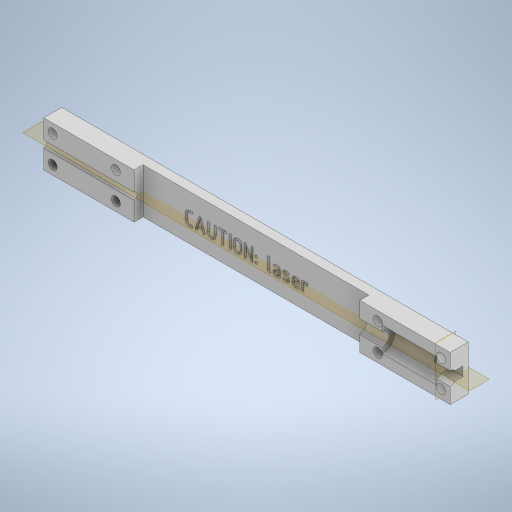
# Autodesk Inventor part: common_bottom
Saved by Autodesk Inventor 2024 (Build 280153000, 153)
## iProperties
Created: 2023-10-30
Part Number: common_bottom
Material: Generic
Document SubType Name: Modeling
Designer: toybox
Density: 1 g/cm^3
Appearance: Default
Author: toybox
Autodesk Inventor part; units mm, degrees
ref_plane "YZ Plane" through (0, 0, 0) normal (1, 0, 0) x (0, 1, 0)
ref_plane "XZ Plane" through (0, 0, 0) normal (0, 1, 0) x (-1, 0, 0)
ref_plane "XY Plane" through (0, 0, 0) normal (0, 0, 1) x (1, 0, 0)
sketch "Sketch1" plane through (0, 0, 0) normal (0, 0, 1) x (1, 0, 0)
  line L0 (-45, 5) -> (45, 5)
  line L1 (45, 5) -> (45, -5)
  line L2 (45, -5) -> (-45, -5)
  line L3 (-45, -5) -> (-45, 5)
  line L4 (-45, 5) -> (45, -5) construction
  line L5 (45, 5) -> (-45, -5) construction
  point P0 (0, 0)
  dimension "d0" = 90
  dimension "d1" = 10
  constraints: 12 end point, 2 midpoint, 2 parallel, 1 horizontal, 1 perpendicular
  measures "d0" distance of L1.end L2.end
  measures "d1" distance of L0.end L1.end
extrude "Extrusion1" add sketch "Sketch1" along normal blind 2
sketch "Sketch4" plane through (0, 0, 2) normal (0, 0, 1) x (1, 0, 0)
  line L0 (45, -5) -> (45, 5) projected
  line L1 (-45, -5) -> (45, -5) projected
  line L2 (45, 5) -> (25, 5)
  line L3 (25, 5) -> (25, -5)
  line L4 (25, -5) -> (45, -5)
  line L5 (45, -5) -> (45, 5)
  line L6 (45, 5) -> (-45, 5) projected
  line L7 (-45, 5) -> (-25, 5)
  line L8 (-25, 5) -> (-25, -5)
  line L9 (-25, -5) -> (-45, -5)
  line L10 (-45, -5) -> (-45, 5)
  point P0 (0, 0)
  dimension "d13" = 20
  dimension "d14" = 20
  constraints: 16 end point, 4 parallel, 2 horizontal, 2 perpendicular, 2 point on line
  measures "d13" distance of L4.end L3.end
  measures "d14" distance of L8.end L9.end
extrude "Extrusion4" add sketch "Sketch4" along normal blind 2 contours L1 L3 L2 L0 | L1 L10 L6 L8
sketch "Sketch5" plane through (0, 0, 4) normal (0, 0, 1) x (1, 0, 0)
  circle A0 centre (43, 3) radius 1
  circle A1 centre (43, -3) radius 1
  circle A2 centre (-43.0005, -3) radius 1
  circle A3 centre (-43.0005, 3) radius 1
  circle A4 centre (-28.9998, -3) radius 1
  circle A5 centre (-28.9998, 3) radius 1
  circle A6 centre (28.9998, -3) radius 1
  circle A7 centre (28.9998, 3) radius 1
  point P0 (0, 0)
  dimension "d17" = 2
  dimension "d18" = 2
  dimension "d19" = 2
  dimension "d20" = 2
  dimension "d22" = 2
  dimension "d23" = 2
  dimension "d24" = 2
  dimension "d25" = 2
  constraints: 8 centre point
  measures "d17" diameter of A0
  measures "d18" diameter of A1
  measures "d19" diameter of A2
  measures "d20" diameter of A3
  measures "d22" diameter of A4
  measures "d23" diameter of A5
  measures "d24" diameter of A6
  measures "d25" diameter of A7
extrude "Extrusion5" cut sketch "Sketch5" against normal through all
sketch "Sketch6" plane through (45, -5, 0) normal (1, 0, 0) x (0, 0, -1)
  line L0 (-4, 0) -> (-4, 10) projected
  circle A0 centre (-4, 5) radius 1.5
  point P0 (0, 5)
  point P1 (-4, 6.5)
  point P2 (-4, 3.5)
  dimension "d28" = 3
  constraints: 1 centre point, 1 midpoint
  measures "d28" diameter of A0
extrude "Extrusion6" cut sketch "Sketch6" against normal blind 20 contours L0 A0 picked at (-3.6883, 5.3909)
sketch "Sketch7" plane through (-45, -5, 0) normal (-1, 0, 0) x (0, 0, 1)
  line L0 (4, 0) -> (4, 10) projected
  circle A0 centre (4, 5) radius 0.75
  point P0 (0, 5)
  dimension "d31" = 1.5
  constraints: 1 centre point, 1 midpoint
  measures "d31" diameter of A0
extrude "Extrusion7" cut sketch "Sketch7" against normal blind 20
ref_plane "Work Plane1" through (42, -5, 0) normal (1, 0, 0) x (0, 0, -1)
sketch "Sketch8" plane through (42, -5, 0) normal (1, 0, 0) x (0, 0, -1)
  arc A0 (-4, 3.5) -> (-4, 6.5) centre (-4, 5) ccw projected
  circle A1 centre (-4, 5) radius 2.7
  point P0 (0, 5)
  dimension "d35" = 5.4
  constraints: 1 centre point, 1 coincident
  measures "d35" diameter of A1
extrude "Extrusion8" cut sketch "Sketch8" against normal blind 12
ref_plane "Work Plane3" through (-45, 0, 0) normal (0, 1, 0) x (1, 0, 0)
sketch "Sketch10" plane through (-45, 0, 0) normal (0, 1, 0) x (1, 0, 0)
  line L0 (90, -2.5) -> (90, -4) projected
  line L1 (90, -4) -> (84, -4)
  line L2 (84, -4) -> (84, -1.2)
  line L3 (84, -1.2) -> (90, -1.2)
  line L4 (90, -1.2) -> (90, -4)
  point P0 (45, 0)
  dimension "d42" = 6
  dimension "d43" = 2.8
  constraints: 8 end point, 2 parallel, 1 horizontal, 1 perpendicular
  measures "d42" distance of L2.end L3.end
  measures "d43" distance of L1.end L2.end
extrude "Extrusion10" cut sketch "Sketch10" along normal mid plane 2
sketch "Sketch11" plane through (0, 0, 2) normal (0, 0, 1) x (1, 0, 0)
  line L0 (-15.8496, 1.3732) -> (11.6508, 1.3732) construction
  line L1 (11.6508, 1.3732) -> (11.6508, -1.6796) construction
  line L2 (11.6508, -1.6796) -> (-15.8496, -1.6796) construction
  line L3 (-15.8496, -1.6796) -> (-15.8496, 1.3732) construction
  spline S0 degree 2 poles (-14.1747, 1.3732) (-13.9787, 1.3732) (-13.9787, 1.18) knots 0 0 0 1 1 1
  spline S1 degree 2 poles (-13.9787, 1.18) (-13.9787, 0.9839) (-14.1747, 0.9839) knots 0 0 0 1 1 1
  line L4 (-14.1747, 0.9839) -> (-14.7685, 0.9839)
  spline S2 degree 2 poles (-14.7685, 0.9839) (-14.9337, 0.9839) (-15.1634, 0.7515) (-15.1634, 0.589) knots 0 0 0 1 2 2 2
  line L5 (-15.1634, 0.589) -> (-15.1634, -0.8925)
  spline S3 degree 2 poles (-15.1634, -0.8925) (-15.1634, -1.0578) (-14.9309, -1.2903) (-14.7685, -1.2903) knots 0 0 0 1 2 2 2
  line L6 (-14.7685, -1.2903) -> (-14.1747, -1.2903)
  spline S4 degree 2 poles (-14.1747, -1.2903) (-13.9787, -1.2903) (-13.9787, -1.4835) knots 0 0 0 1 1 1
  spline S5 degree 2 poles (-13.9787, -1.4835) (-13.9787, -1.6796) (-14.1747, -1.6796) knots 0 0 0 1 1 1
  line L7 (-14.1747, -1.6796) -> (-14.7685, -1.6796)
  spline S6 degree 2 poles (-14.7685, -1.6796) (-15.0962, -1.6796) (-15.5555, -1.2202) (-15.5555, -0.8925) knots 0 0 0 1 2 2 2
  line L8 (-15.5555, -0.8925) -> (-15.5555, 0.589)
  spline S7 degree 2 poles (-15.5555, 0.589) (-15.5555, 0.9139) (-15.0962, 1.3732) (-14.7685, 1.3732) knots 0 0 0 1 2 2 2
  line L9 (-14.7685, 1.3732) -> (-14.1747, 1.3732)
  spline S8 degree 2 poles (-11.2732, -1.4835) (-11.2732, -1.6796) (-11.4692, -1.6796) knots 0 0 0 1 1 1
  spline S9 degree 2 poles (-11.4692, -1.6796) (-11.6121, -1.6796) (-11.6541, -1.5479) knots 0 0 0 1 1 1
  line L10 (-11.6541, -1.5479) -> (-11.8585, -0.9402)
  line L11 (-11.8585, -0.9402) -> (-12.8556, -0.9402)
  line L12 (-12.8556, -0.9402) -> (-13.0572, -1.5479)
  spline S10 degree 2 poles (-13.0572, -1.5479) (-13.102, -1.6796) (-13.2449, -1.6796) knots 0 0 0 1 1 1
  spline S11 degree 2 poles (-13.2449, -1.6796) (-13.4381, -1.6796) (-13.4381, -1.4835) knots 0 0 0 1 1 1
  spline S12 degree 2 poles (-13.4381, -1.4835) (-13.4381, -1.4499) (-13.4297, -1.4219) knots 0 0 0 1 1 1
  line L13 (-13.4297, -1.4219) -> (-12.5503, 1.222)
  spline S13 degree 2 poles (-12.5503, 1.222) (-12.4999, 1.3704) (-12.357, 1.3704) knots 0 0 0 1 1 1
  spline S14 degree 2 poles (-12.357, 1.3704) (-12.2142, 1.3704) (-12.1666, 1.2248) knots 0 0 0 1 1 1
  line L14 (-12.1666, 1.2248) -> (-11.2816, -1.4219)
  spline S15 degree 2 poles (-11.2816, -1.4219) (-11.2732, -1.4527) (-11.2732, -1.4835) knots 0 0 0 1 1 1
  line L15 (-12.357, 0.6619) -> (-12.7436, -0.5509)
  line L16 (-12.7436, -0.5509) -> (-11.9677, -0.5509)
  line L17 (-11.9677, -0.5509) -> (-12.357, 0.6619)
  line L18 (-8.8505, 1.1772) -> (-8.8505, -0.7441)
  spline S16 degree 2 poles (-8.8505, -0.7441) (-8.8505, -1.1334) (-9.3967, -1.6796) (-9.7832, -1.6796) knots 0 0 0 1 2 2 2
  spline S17 degree 2 poles (-9.7832, -1.6796) (-10.1725, -1.6796) (-10.7186, -1.1334) (-10.7186, -0.7441) knots 0 0 0 1 2 2 2
  line L19 (-10.7186, -0.7441) -> (-10.7186, 1.1772)
  spline S18 degree 2 poles (-10.7186, 1.1772) (-10.7186, 1.3704) (-10.5226, 1.3704) knots 0 0 0 1 1 1
  spline S19 degree 2 poles (-10.5226, 1.3704) (-10.3265, 1.3704) (-10.3265, 1.1772) knots 0 0 0 1 1 1
  line L20 (-10.3265, 1.1772) -> (-10.3265, -0.7441)
  spline S20 degree 2 poles (-10.3265, -0.7441) (-10.3265, -0.9738) (-10.0128, -1.2903) (-9.7832, -1.2903) knots 0 0 0 1 2 2 2
  spline S21 degree 2 poles (-9.7832, -1.2903) (-9.5563, -1.2903) (-9.2426, -0.9738) (-9.2426, -0.7441) knots 0 0 0 1 2 2 2
  line L21 (-9.2426, -0.7441) -> (-9.2426, 1.1772)
  spline S22 degree 2 poles (-9.2426, 1.1772) (-9.2426, 1.3704) (-9.0466, 1.3704) knots 0 0 0 1 1 1
  spline S23 degree 2 poles (-9.0466, 1.3704) (-8.8505, 1.3704) (-8.8505, 1.1772) knots 0 0 0 1 1 1
  spline S24 degree 2 poles (-8.3016, 1.18) (-8.3016, 1.3732) (-8.1055, 1.3732) knots 0 0 0 1 1 1
  line L22 (-8.1055, 1.3732) -> (-6.6267, 1.3732)
  spline S25 degree 2 poles (-6.6267, 1.3732) (-6.4307, 1.3732) (-6.4307, 1.18) knots 0 0 0 1 1 1
  spline S26 degree 2 poles (-6.4307, 1.18) (-6.4307, 0.9839) (-6.6267, 0.9839) knots 0 0 0 1 1 1
  line L23 (-6.6267, 0.9839) -> (-7.1701, 0.9839)
  line L24 (-7.1701, 0.9839) -> (-7.1701, -1.4835)
  spline S27 degree 2 poles (-7.1701, -1.4835) (-7.1701, -1.6796) (-7.3661, -1.6796) knots 0 0 0 1 1 1
  spline S28 degree 2 poles (-7.3661, -1.6796) (-7.5622, -1.6796) (-7.5622, -1.4835) knots 0 0 0 1 1 1
  line L25 (-7.5622, -1.4835) -> (-7.5622, 0.9839)
  line L26 (-7.5622, 0.9839) -> (-8.1055, 0.9839)
  spline S29 degree 2 poles (-8.1055, 0.9839) (-8.3016, 0.9839) (-8.3016, 1.18) knots 0 0 0 1 1 1
  spline S30 degree 2 poles (-5.6913, -1.6796) (-5.8874, -1.6796) (-5.8874, -1.4835) knots 0 0 0 1 1 1
  line L27 (-5.8874, -1.4835) -> (-5.8874, 1.1772)
  spline S31 degree 2 poles (-5.8874, 1.1772) (-5.8874, 1.3704) (-5.6913, 1.3704) knots 0 0 0 1 1 1
  spline S32 degree 2 poles (-5.6913, 1.3704) (-5.4952, 1.3704) (-5.4952, 1.1772) knots 0 0 0 1 1 1
  line L28 (-5.4952, 1.1772) -> (-5.4952, -1.4835)
  spline S33 degree 2 poles (-5.4952, -1.4835) (-5.4952, -1.6796) (-5.6913, -1.6796) knots 0 0 0 1 1 1
  spline S34 degree 2 poles (-3.109, -0.7441) (-3.109, -1.1306) (-3.6552, -1.6796) (-4.0417, -1.6796) knots 0 0 0 1 2 2 2
  spline S35 degree 2 poles (-4.0417, -1.6796) (-4.431, -1.6796) (-4.9771, -1.1334) (-4.9771, -0.7441) knots 0 0 0 1 2 2 2
  line L29 (-4.9771, -0.7441) -> (-4.9771, 0.4406)
  spline S36 degree 2 poles (-4.9771, 0.4406) (-4.9771, 0.8271) (-4.431, 1.3732) (-4.0417, 1.3732) knots 0 0 0 1 2 2 2
  spline S37 degree 2 poles (-4.0417, 1.3732) (-3.6524, 1.3732) (-3.109, 0.8271) (-3.109, 0.4406) knots 0 0 0 1 2 2 2
  line L30 (-3.109, 0.4406) -> (-3.109, -0.7441)
  line L31 (-3.5011, -0.7441) -> (-3.5011, 0.4406)
  spline S38 degree 2 poles (-3.5011, 0.4406) (-3.5011, 0.6675) (-3.8148, 0.9839) (-4.0417, 0.9839) knots 0 0 0 1 2 2 2
  spline S39 degree 2 poles (-4.0417, 0.9839) (-4.2713, 0.9839) (-4.585, 0.6675) (-4.585, 0.4406) knots 0 0 0 1 2 2 2
  line L32 (-4.585, 0.4406) -> (-4.585, -0.7441)
  spline S40 degree 2 poles (-4.585, -0.7441) (-4.585, -0.9738) (-4.2713, -1.2903) (-4.0417, -1.2903) knots 0 0 0 1 2 2 2
  spline S41 degree 2 poles (-4.0417, -1.2903) (-3.8148, -1.2903) (-3.5011, -0.9738) (-3.5011, -0.7441) knots 0 0 0 1 2 2 2
  line L33 (-1.0841, -0.8645) -> (-1.0841, 1.1772)
  spline S42 degree 2 poles (-1.0841, 1.1772) (-1.0841, 1.3704) (-0.888, 1.3704) knots 0 0 0 1 1 1
  spline S43 degree 2 poles (-0.888, 1.3704) (-0.692, 1.3704) (-0.692, 1.1772) knots 0 0 0 1 1 1
  line L34 (-0.692, 1.1772) -> (-0.692, -1.4835)
  spline S44 degree 2 poles (-0.692, -1.4835) (-0.692, -1.6796) (-0.888, -1.6796) knots 0 0 0 1 1 1
  spline S45 degree 2 poles (-0.888, -1.6796) (-1.0085, -1.6796) (-1.0617, -1.5815) knots 0 0 0 1 1 1
  line L35 (-1.0617, -1.5815) -> (-2.168, 0.561)
  line L36 (-2.168, 0.561) -> (-2.168, -1.4835)
  spline S46 degree 2 poles (-2.168, -1.4835) (-2.168, -1.6796) (-2.364, -1.6796) knots 0 0 0 1 1 1
  spline S47 degree 2 poles (-2.364, -1.6796) (-2.5601, -1.6796) (-2.5601, -1.4835) knots 0 0 0 1 1 1
  line L37 (-2.5601, -1.4835) -> (-2.5601, 1.1772)
  spline S48 degree 2 poles (-2.5601, 1.1772) (-2.5601, 1.3704) (-2.364, 1.3704) knots 0 0 0 1 1 1
  spline S49 degree 2 poles (-2.364, 1.3704) (-2.2492, 1.3704) (-2.2016, 1.2864) knots 0 0 0 1 1 1
  line L38 (-2.2016, 1.2864) -> (-1.0841, -0.8645)
  spline S50 degree 2 poles (-0.1458, -1.1866) (-0.1458, -0.9962) (0.0502, -0.9962) knots 0 0 0 1 1 1
  spline S51 degree 2 poles (0.0502, -0.9962) (0.2463, -0.9962) (0.2463, -1.1866) knots 0 0 0 1 1 1
  line L39 (0.2463, -1.1866) -> (0.2463, -1.3351)
  spline S52 degree 2 poles (0.2463, -1.3351) (0.2463, -1.5311) (0.0502, -1.5311) knots 0 0 0 1 1 1
  spline S53 degree 2 poles (0.0502, -1.5311) (-0.1458, -1.5311) (-0.1458, -1.3351) knots 0 0 0 1 1 1
  line L40 (-0.1458, -1.3351) -> (-0.1458, -1.1866)
  spline S54 degree 2 poles (-0.1458, -0.0047) (-0.1458, 0.1885) (0.0502, 0.1885) knots 0 0 0 1 1 1
  spline S55 degree 2 poles (0.0502, 0.1885) (0.2463, 0.1885) (0.2463, -0.0047) knots 0 0 0 1 1 1
  line L41 (0.2463, -0.0047) -> (0.2463, -0.1532)
  spline S56 degree 2 poles (0.2463, -0.1532) (0.2463, -0.3464) (0.0502, -0.3464) knots 0 0 0 1 1 1
  spline S57 degree 2 poles (0.0502, -0.3464) (-0.1458, -0.3464) (-0.1458, -0.1532) knots 0 0 0 1 1 1
  line L42 (-0.1458, -0.1532) -> (-0.1458, -0.0047)
  spline S58 degree 2 poles (2.5765, 1.1772) (2.5765, 1.3704) (2.7725, 1.3704) knots 0 0 0 1 1 1
  spline S59 degree 2 poles (2.7725, 1.3704) (2.9686, 1.3704) (2.9686, 1.1772) knots 0 0 0 1 1 1
  line L43 (2.9686, 1.1772) -> (2.9686, -1.1894)
  spline S60 degree 2 poles (2.9686, -1.1894) (2.9686, -1.2678) (3.2654, -1.3351) (3.2654, -1.4835) knots 0 0 0 1 2 2 2
  spline S61 degree 2 poles (3.2654, -1.4835) (3.2654, -1.6796) (3.0694, -1.6796) knots 0 0 0 1 1 1
  spline S62 degree 2 poles (3.0694, -1.6796) (2.8481, -1.6796) (2.5765, -1.4191) (2.5765, -1.1894) knots 0 0 0 1 2 2 2
  line L44 (2.5765, -1.1894) -> (2.5765, 1.1772)
  spline S63 degree 2 poles (4.4278, -1.6796) (4.1561, -1.6796) (3.7864, -1.3099) (3.7864, -1.0382) knots 0 0 0 1 2 2 2
  spline S64 degree 2 poles (3.7864, -1.0382) (3.7864, -0.8673) (3.8732, -0.7189) knots 0 0 0 1 1 1
  spline S65 degree 2 poles (3.8732, -0.7189) (4.0525, -0.4024) (4.4278, -0.4024) knots 0 0 0 1 1 1
  line L45 (4.4278, -0.4024) -> (4.9711, -0.4024)
  line L46 (4.9711, -0.4024) -> (4.9711, -0.1504)
  spline S66 degree 2 poles (4.9711, -0.1504) (4.9711, -0.0467) (4.8283, 0.0961) (4.7218, 0.0961) knots 0 0 0 1 2 2 2
  line L47 (4.7218, 0.0961) -> (4.1309, 0.0961)
  spline S67 degree 2 poles (4.1309, 0.0961) (3.9348, 0.0961) (3.9348, 0.2922) knots 0 0 0 1 1 1
  spline S68 degree 2 poles (3.9348, 0.2922) (3.9348, 0.4854) (4.1309, 0.4854) knots 0 0 0 1 1 1
  line L48 (4.1309, 0.4854) -> (4.7218, 0.4854)
  spline S69 degree 2 poles (4.7218, 0.4854) (4.9907, 0.4854) (5.3632, 0.1157) (5.3632, -0.1504) knots 0 0 0 1 2 2 2
  line L49 (5.3632, -0.1504) -> (5.3632, -1.4835)
  spline S70 degree 2 poles (5.3632, -1.4835) (5.3632, -1.6796) (5.1671, -1.6796) knots 0 0 0 1 1 1
  line L50 (5.1671, -1.6796) -> (4.4278, -1.6796)
  line L51 (4.9711, -0.7917) -> (4.4278, -0.7917)
  spline S71 degree 2 poles (4.4278, -0.7917) (4.3241, -0.7917) (4.1785, -0.9374) (4.1785, -1.0382) knots 0 0 0 1 2 2 2
  spline S72 degree 2 poles (4.1785, -1.0382) (4.1785, -1.1418) (4.3269, -1.2903) (4.4278, -1.2903) knots 0 0 0 1 2 2 2
  line L52 (4.4278, -1.2903) -> (4.9711, -1.2903)
  line L53 (4.9711, -1.2903) -> (4.9711, -0.7917)
  spline S73 degree 2 poles (7.0857, -1.1138) (7.0857, -1.0018) (6.9876, -0.9542) knots 0 0 0 1 1 1
  line L54 (6.9876, -0.9542) -> (6.2286, -0.5901)
  spline S74 degree 2 poles (6.2286, -0.5901) (5.9037, -0.4332) (5.9037, -0.0775) knots 0 0 0 1 1 1
  spline S75 degree 2 poles (5.9037, -0.0775) (5.9037, 0.2025) (6.1334, 0.3538) knots 0 0 0 1 1 1
  spline S76 degree 2 poles (6.1334, 0.3538) (6.3267, 0.4826) (6.6151, 0.4826) knots 0 0 0 1 1 1
  spline S77 degree 2 poles (6.6151, 0.4826) (6.9568, 0.4826) (7.2285, 0.3118) knots 0 0 0 1 1 1
  spline S78 degree 2 poles (7.2285, 0.3118) (7.3293, 0.2474) (7.3293, 0.1437) knots 0 0 0 1 1 1
  spline S79 degree 2 poles (7.3293, 0.1437) (7.3293, 0.0625) (7.2145, -0.0523) (7.1333, -0.0523) knots 0 0 0 1 2 2 2
  spline S80 degree 2 poles (7.1333, -0.0523) (7.08, -0.0523) (7.0156, -0.0131) knots 0 0 0 1 1 1
  spline S81 degree 2 poles (7.0156, -0.0131) (6.8392, 0.0933) (6.6151, 0.0933) knots 0 0 0 1 1 1
  spline S82 degree 2 poles (6.6151, 0.0933) (6.293, 0.0933) (6.293, -0.0775) knots 0 0 0 1 1 1
  spline S83 degree 2 poles (6.293, -0.0775) (6.293, -0.1924) (6.3883, -0.2372) knots 0 0 0 1 1 1
  line L55 (6.3883, -0.2372) -> (7.1529, -0.6069)
  spline S84 degree 2 poles (7.1529, -0.6069) (7.4778, -0.7637) (7.4778, -1.1138) knots 0 0 0 1 1 1
  spline S85 degree 2 poles (7.4778, -1.1138) (7.4778, -1.4107) (7.2425, -1.5591) knots 0 0 0 1 1 1
  spline S86 degree 2 poles (7.2425, -1.5591) (7.0492, -1.6796) (6.7496, -1.6796) knots 0 0 0 1 1 1
  spline S87 degree 2 poles (6.7496, -1.6796) (6.3098, -1.6796) (6.0102, -1.5087) knots 0 0 0 1 1 1
  spline S88 degree 2 poles (6.0102, -1.5087) (5.9037, -1.4499) (5.9037, -1.3351) knots 0 0 0 1 1 1
  spline S89 degree 2 poles (5.9037, -1.3351) (5.9037, -1.2566) (6.0158, -1.1418) (6.097, -1.1418) knots 0 0 0 1 2 2 2
  spline S90 degree 2 poles (6.097, -1.1418) (6.1362, -1.1418) (6.1558, -1.1502) knots 0 0 0 1 1 1
  spline S91 degree 2 poles (6.1558, -1.1502) (6.237, -1.1866) (6.3855, -1.2398) knots 0 0 0 1 1 1
  spline S92 degree 2 poles (6.3855, -1.2398) (6.5703, -1.2903) (6.758, -1.2903) knots 0 0 0 1 1 1
  spline S93 degree 2 poles (6.758, -1.2903) (7.0857, -1.2903) (7.0857, -1.1138) knots 0 0 0 1 1 1
  line L56 (8.4076, -0.7917) -> (8.4076, -1.0382)
  spline S94 degree 2 poles (8.4076, -1.0382) (8.4076, -1.1418) (8.556, -1.2903) (8.6569, -1.2903) knots 0 0 0 1 2 2 2
  line L57 (8.6569, -1.2903) -> (9.3963, -1.2903)
  spline S95 degree 2 poles (9.3963, -1.2903) (9.5923, -1.2903) (9.5923, -1.4835) knots 0 0 0 1 1 1
  spline S96 degree 2 poles (9.5923, -1.4835) (9.5923, -1.6796) (9.3963, -1.6796) knots 0 0 0 1 1 1
  line L58 (9.3963, -1.6796) -> (8.6569, -1.6796)
  spline S97 degree 2 poles (8.6569, -1.6796) (8.3852, -1.6796) (8.0155, -1.3099) (8.0155, -1.041) knots 0 0 0 1 2 2 2
  line L59 (8.0155, -1.041) -> (8.0155, -0.3016)
  spline S98 degree 2 poles (8.0155, -0.3016) (8.0155, 0.0233) (8.4748, 0.4826) (8.8025, 0.4826) knots 0 0 0 1 2 2 2
  spline S99 degree 2 poles (8.8025, 0.4826) (9.1358, 0.4826) (9.5923, 0.0289) (9.5923, -0.3016) knots 0 0 0 1 2 2 2
  line L60 (9.5923, -0.3016) -> (9.5923, -0.7917)
  line L61 (9.5923, -0.7917) -> (8.4076, -0.7917)
  spline S100 degree 2 poles (8.8025, 0.0961) (8.6401, 0.0961) (8.4076, -0.1363) (8.4076, -0.2988) knots 0 0 0 1 2 2 2
  line L62 (8.4076, -0.2988) -> (8.4076, -0.4024)
  line L63 (8.4076, -0.4024) -> (9.2002, -0.4024)
  line L64 (9.2002, -0.4024) -> (9.2002, -0.2988)
  spline S101 degree 2 poles (9.2002, -0.2988) (9.2002, -0.1363) (8.9677, 0.0961) (8.8025, 0.0961) knots 0 0 0 1 2 2 2
  spline S102 degree 2 poles (10.13, 0.2922) (10.13, 0.4854) (10.3261, 0.4854) knots 0 0 0 1 1 1
  line L65 (10.3261, 0.4854) -> (11.2139, 0.4854)
  spline S103 degree 2 poles (11.2139, 0.4854) (11.41, 0.4854) (11.41, 0.2922) knots 0 0 0 1 1 1
  line L66 (11.41, 0.2922) -> (11.41, -0.0047)
  spline S104 degree 2 poles (11.41, -0.0047) (11.41, -0.2008) (11.2139, -0.2008) knots 0 0 0 1 1 1
  spline S105 degree 2 poles (11.2139, -0.2008) (11.0179, -0.2008) (11.0179, -0.0047) knots 0 0 0 1 1 1
  line L67 (11.0179, -0.0047) -> (11.0179, 0.0961)
  line L68 (11.0179, 0.0961) -> (10.5222, 0.0961)
  line L69 (10.5222, 0.0961) -> (10.5222, -1.4835)
  spline S106 degree 2 poles (10.5222, -1.4835) (10.5222, -1.6796) (10.3261, -1.6796) knots 0 0 0 1 1 1
  spline S107 degree 2 poles (10.3261, -1.6796) (10.13, -1.6796) (10.13, -1.4835) knots 0 0 0 1 1 1
  line L70 (10.13, -1.4835) -> (10.13, 0.2922)
  point P0 (0, 0)
  constraints: 2 other
extrude "Extrusion11" cut sketch "Sketch11" against normal blind 0.5
body "Solid1"
